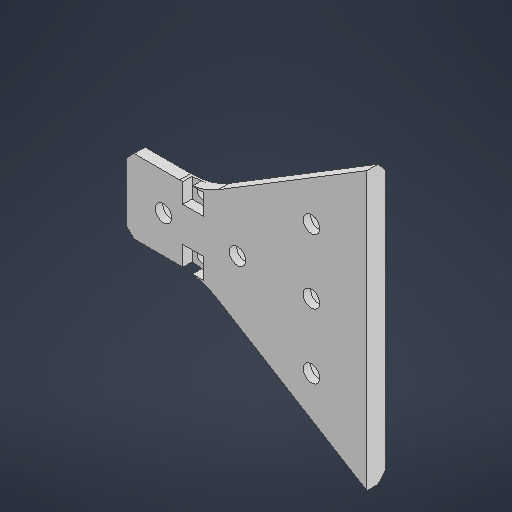
# Autodesk Inventor part: Y Axis Holder
Saved by Autodesk Inventor 2025.1 (Build 291241000, 241)
## iProperties
Created: 2025-02-22
Part Number: Y Axis Holder
Material: Generic
Document SubType Name: Modeling
Designer: jerem
Density: 1 g/cm^3
Appearance: Default
Author: jerem
## iProperties of the stored document Y Axis Holder_3DPrint.ipt
Created: 2025-02-22
Part Number: Y Axis Holder_3DPrint
Material: Generic
Document SubType Name: Modeling
Designer: jerem
Density: 1 g/cm^3
Appearance: Default
Author: jerem
Autodesk Inventor part; units mm, degrees
ref_plane "YZ Plane" through (0, 0, 0) normal (1, 0, 0) x (0, 1, 0)
ref_plane "XZ Plane" through (0, 0, 0) normal (0, 1, 0) x (-1, 0, 0)
ref_plane "XY Plane" through (0, 0, 0) normal (0, 0, 1) x (1, 0, 0)
sketch "Sketch1" plane through (0, 0, 0) normal (0, 0, 1) x (1, 0, 0)
  line L0 (0, 0) -> (-50, 0) construction
  line L1 (-50, 0) -> (-50, 10)
  line L2 (-50, 0) -> (-50, -10)
  line L3 (-50, -10) -> (-30, -10)
  line L4 (-30, -10) -> (15, -37.5)
  line L5 (-50, 10) -> (-30, 10)
  line L6 (-30, 10) -> (15, 37.5)
  line L7 (15, 37.5) -> (15, -37.5)
  line L8 (0, 0) -> (15, 0) construction
  line L9 (0, 17.5) -> (0, -17.5) construction
  point P0 (-40, 0)
  point P1 (-20, 0)
  dimension "d0" = 20
  dimension "d1" = 65
  dimension "d2" = 50
  dimension "d4" = 20
  dimension "d5" = 75
  dimension "d6" = 35
  dimension "d9" = 40
  dimension "d41" = 20
  constraints: 20 end point, 3 coincident, 3 equal length, 3 vertical, 2 horizontal, 2 midpoint, 2 perpendicular, 2 point on line
  measures "d0" distance between parallel lines of L3 L5
  measures "d1" distance of L8.end L0.end
  measures "d2" distance between parallel lines of L1 L9
  measures "d4" distance of L1.end L5.end
  measures "d5" distance of L6.end L4.end
  measures "d6" distance of L9.end L9.start
  measures "d9" distance of L0.start point (-40, 0)
  measures "d41" distance of L0.start point (-20, 0)
extrude "Extrusion1" add sketch "Sketch1" along normal blind 5
hole "Hole1" at (0, 17.5, 0) at (0, -17.5, 0) at (-40, 0, 0) at (0, 0, 0) at (-20, 0, 0) direction (0, 0, 1) diameter 4.5 end through all counterbore diameter 8 counterbore depth 3
fillet "Fillet1" radius 20 2 edges at (-30, 10, 2.5) (-30, -10, 2.5)
chamfer "Chamfer1" distance 2 angle 45 2 edges at (-50, 10, 2.5) (-50, -10, 2.5)
sketch "Sketch2" plane through (0, 0, 0) normal (0, 0, -1) x (-1, 0, 0)
  line L0 (50, -8) -> (48, -10) projected
  line L1 (50, 8) -> (50, -8) projected
  line L2 (48, 10) -> (50, 8) projected
  line L3 (35.6273, 10) -> (48, 10) projected
  arc A0 (25.1983, 12.9344) -> (35.6273, 10) centre (35.6273, 30) ccw projected
  line L4 (-15, 37.5) -> (25.1983, 12.9344) projected
  line L5 (-15, -37.5) -> (-15, 37.5) projected
  line L6 (25.1983, -12.9344) -> (-15, -37.5) projected
  arc A1 (35.6273, -10) -> (25.1983, -12.9344) centre (35.6273, -30) ccw projected
  line L7 (48, -10) -> (35.6273, -10) projected
  circle A2 centre (0, 0) radius 4 projected
  circle A3 centre (40, 0) radius 4 projected
  circle A4 centre (0, -17.5) radius 4 projected
  circle A5 centre (0, 17.5) radius 4 projected
  line L8 (32, 7.5) -> (32, -7.5) construction
  line L9 (50, 0) -> (32, 0) construction
  circle A6 centre (32, 7.5) radius 1.5
  circle A7 centre (32, -7.5) radius 1.5
  line L10 (29, 4) -> (32, 4)
  line L11 (32, 4) -> (32, -4)
  line L12 (32, -4) -> (29, -4)
  line L13 (29, -4) -> (29, 4)
  line L14 (50, 4) -> (47, 4)
  line L15 (47, 4) -> (47, -4)
  line L16 (47, -4) -> (50, -4)
  line L17 (50, -4) -> (50, 4)
  line L18 (50, 8) -> (50, -8) projected
  point P0 (32, 0)
  point P1 (47, 0)
  dimension "d24" = 18
  dimension "d25" = 15
  dimension "d26" = 3
  dimension "d27" = 3
  dimension "d30" = 3
  dimension "d31" = 3
  dimension "d32" = 8
  dimension "d33" = 8
  dimension "d34" = 3
  constraints: 20 end point, 6 midpoint, 4 parallel, 3 horizontal, 2 centre point, 2 coincident, 2 perpendicular, 2 point on line, 1 vertical
  measures "d24" distance of L9.start L9.end
  measures "d25" distance of L8.start L8.end
  measures "d26" diameter of A6
  measures "d27" diameter of A7
  measures "d30" distance between parallel lines of L8 L13
  measures "d31" distance of L10.start L10.end
  measures "d32" distance of L12.end L10.start
  measures "d33" distance of L14.end L15.end
  measures "d34" distance of L14.start L14.end
extrude "Extrusion2" cut sketch "Sketch2" against normal through all contours A6 | A7
chamfer "Chamfer2" distance 2 angle 45 6 edges at (-41.8137, 10, 0) (-30.2103, 10.7476, 0) (-5.0992, 25.2172, 0) (-30.2103, -10.7476, 0) (-5.0992, -25.2172, 0) (-41.8137, -10, 0)
sketch "Sketch3" plane through (0, 0, 5) normal (0, 0, 1) x (1, 0, 0)
  circle A0 centre (-32, 7.5) radius 1.5 projected
  circle A1 centre (-32, -7.5) radius 1.5 projected
  line L0 (-29.2, 4.7) -> (-34.8, 4.7)
  line L1 (-34.8, 4.7) -> (-34.8, 10.3)
  line L2 (-34.8, 10.3) -> (-29.2, 10.3)
  line L3 (-29.2, 10.3) -> (-29.2, 4.7)
  line L4 (-29.2, 4.7) -> (-34.8, 10.3) construction
  line L5 (-34.8, 4.7) -> (-29.2, 10.3) construction
  line L6 (-29.2, -10.3) -> (-34.8, -10.3)
  line L7 (-34.8, -10.3) -> (-34.8, -4.7)
  line L8 (-34.8, -4.7) -> (-29.2, -4.7)
  line L9 (-29.2, -4.7) -> (-29.2, -10.3)
  line L10 (-29.2, -10.3) -> (-34.8, -4.7) construction
  line L11 (-34.8, -10.3) -> (-29.2, -4.7) construction
  point P0 (0, 0)
  dimension "d37" = 5.6
  dimension "d38" = 5.6
  constraints: 24 end point, 4 midpoint, 4 parallel, 2 horizontal, 2 perpendicular, 1 collinear, 1 point on line
  measures "d37" distance of L1.end L2.end
  measures "d38" distance of L0.end L1.end
extrude "Extrusion4" cut sketch "Sketch3" against normal blind 2.5
equation "\"d27\" = d26"
body "Solid1"
